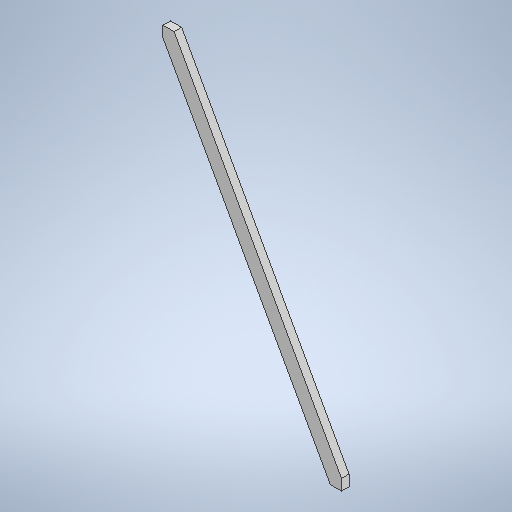
# Autodesk Inventor part: Support - Left
Saved by Autodesk Inventor 2025.2 (Build 292293000, 293)
## iProperties
Created: 2025-02-17
Part Number: Support - Left
Material: Generic
Document SubType Name: Modeling
Designer: baolo
Density: 1 g/cm^3
Appearance: Default
Author: baolo
Autodesk Inventor part; units mm, degrees
ref_plane "YZ Plane" through (0, 0, 0) normal (1, 0, 0) x (0, 1, 0)
ref_plane "XZ Plane" through (0, 0, 0) normal (0, 1, 0) x (-1, 0, 0)
ref_plane "XY Plane" through (0, 0, 0) normal (0, 0, 1) x (1, 0, 0)
sketch "Sketch1" plane through (0, 0, 0) normal (0, 0, 1) x (1, 0, 0)
  line L0 (-284.5068, 0) -> (47.4178, 0) construction
  line L1 (-14.7186, 14.7186) -> (0, 14.7186) construction
  line L2 (0, 14.7186) -> (0, 0)
  line L3 (0, 0) -> (-14.7186, 0)
  line L4 (-14.7186, 0) -> (-14.7186, 14.7186) construction
  line L5 (-14.7186, 14.7186) -> (0, 0) construction
  line L6 (0, 14.7186) -> (-14.7186, 0) construction
  line L7 (-237.089, 417.3593) -> (-222.3704, 417.3593)
  line L8 (-222.3704, 417.3593) -> (-222.3704, 402.6407) construction
  line L9 (-222.3704, 402.6407) -> (-237.089, 402.6407) construction
  line L10 (-237.089, 402.6407) -> (-237.089, 417.3593)
  line L11 (-237.089, 417.3593) -> (-222.3704, 402.6407) construction
  line L12 (-222.3704, 417.3593) -> (-237.089, 402.6407) construction
  line L13 (-237.089, 402.6407) -> (-14.7186, 0)
  line L14 (-222.3704, 417.3593) -> (0, 14.7186)
  point P0 (-7.3593, 7.3593)
  point P1 (-229.7297, 410)
  dimension "d16" = 480
  dimension "d17" = 20
  dimension "d18" = 410
  constraints: 28 end point, 4 midpoint, 4 parallel, 3 equal length, 2 horizontal, 2 perpendicular
  measures "d16" distance of L2.end L7.start
  measures "d17" distance between parallel lines of L13 L14
  measures "d18" distance from line of L0 point (-229.73, 410)
extrude "Extrusion1" add sketch "Sketch1" along normal mid plane 10
body "Solid1"
